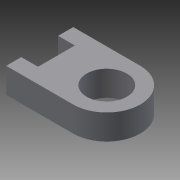
# Autodesk Inventor part: 零件2
Saved by Autodesk Inventor 2014 (Build 180170000, 170)
## iProperties
Created: 2018-10-26
Part Number: 零件2
Material: 常规
Document SubType Name: Modeling
Designer: Administrator
Density: 1 g/cm^3
Appearance: 默认
Author: Administrator
Autodesk Inventor part; units mm, degrees
ref_plane "YZ Plane" through (0, 0, 0) normal (1, 0, 0) x (0, 1, 0)
ref_plane "XZ Plane" through (0, 0, 0) normal (0, 1, 0) x (-1, 0, 0)
ref_plane "XY Plane" through (0, 0, 0) normal (0, 0, 1) x (1, 0, 0)
sketch "草图1" plane through (0, 0, 0) normal (0, 0, 1) x (1, 0, 0)
  circle A0 centre (0, 0) radius 12
  arc A1 (0, -20) -> (0, 20) centre (0, 0) ccw
  line L0 (-41.8118, 0) -> (36.5157, 0)
  line L1 (0, -20) -> (-40, -20)
  line L2 (0, 20) -> (-40, 20)
  line L3 (-40, 11) -> (-30, 11)
  line L4 (-30, -11) -> (-30, 11)
  line L5 (-40, -11) -> (-30, -11)
  line L6 (-40, -20) -> (-40, -11)
  line L7 (-40, 11) -> (-40, 20)
  dimension "d0" = 40
  dimension "d1" = 20
  dimension "d2" = 24
  dimension "d3" = 10
  dimension "d4" = 22
  constraints: 16 end point, 3 parallel, 3 perpendicular, 2 centre point, 2 point on circle, 2 tangent, 1 coincident, 1 collinear, 1 concentric, 1 horizontal, 2 other
  measures "d0" distance of L2.start L2.end
  measures "d1" radius of A1
  measures "d2" diameter of A0
  measures "d3" distance of L5.start L4.start
  measures "d4" distance of L4.start L3.end
extrude "拉伸1" add sketch "草图1" along normal blind 15 contours L0 A1 L1 L6 L5 L4 A0 | A0 L0 L4 L3 L7 L2 A1
